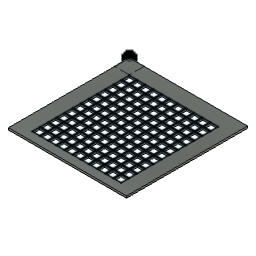
WordClock Raster (Autodesk Fusion 360 design; units mm, degrees)
Autodesk Fusion 360 part; units mm, degrees
sketch "Skizze1" plane through (0, 0, 0) normal (0, 0, 1) x (1, 0, 0)
  line L0 (-74.7669, 75.1961) -> (165.2331, 75.1961)
  line L1 (165.2331, 75.1961) -> (165.2331, -170.8039)
  line L2 (165.2331, -170.8039) -> (-74.7669, -170.8039)
  line L3 (-74.7669, -170.8039) -> (-74.7669, 75.1961)
  dimension "d1" = 240
  dimension "d2" = 246
  constraint horizontal L0
  constraint vertical L1
  constraint horizontal L2
  constraint vertical L3
  measures "d1" distance of L0.start L0.end
  measures "d2" distance of L0.start L2.end
extrude "Extrusion1" add sketch "Skizze1" along normal blind 4
sketch "Skizze2" plane through (0, 0, 4) normal (0, 0, 1) x (-1, 0, 0)
  line L0 (74.7669, 170.8039) -> (-165.2331, 170.8039)
  line L1 (-165.2331, 170.8039) -> (-165.2331, -75.1961)
  line L2 (-165.2331, -75.1961) -> (74.7669, -75.1961)
  line L3 (74.7669, -75.1961) -> (74.7669, 170.8039)
  line L4 (74.7669, -75.1961) -> (44.7989, -75.1961) construction
  line L5 (44.7989, -75.1961) -> (44.7989, -44.9311) construction
  line L6 (44.7989, -44.9311) -> (74.7669, -44.9311) construction
  line L7 (74.7669, -44.9311) -> (74.7669, -75.1961) construction
  line L8 (44.7989, -44.9311) -> (43.7989, -44.9311) construction
  line L9 (43.7989, -44.9311) -> (43.7989, -43.9311) construction
  line L10 (43.7989, -43.9311) -> (44.7989, -43.9311) construction
  line L11 (44.7989, -43.9311) -> (44.7989, -44.9311) construction
  line L12 (43.7989, -43.9311) -> (29.1989, -43.9311)
  line L13 (29.1989, -43.9311) -> (29.1989, -29.3311)
  line L14 (29.1989, -29.3311) -> (43.7989, -29.3311)
  line L15 (43.7989, -29.3311) -> (43.7989, -43.9311)
  line L16 (12.5989, -43.9311) -> (12.5989, -29.3311)
  line L17 (12.5989, -29.3311) -> (27.1989, -29.3311)
  line L18 (27.1989, -29.3311) -> (27.1989, -43.9311)
  line L19 (27.1989, -43.9311) -> (12.5989, -43.9311)
  line L20 (-4.0011, -43.9311) -> (-4.0011, -29.3311)
  line L21 (-4.0011, -29.3311) -> (10.5989, -29.3311)
  line L22 (10.5989, -29.3311) -> (10.5989, -43.9311)
  line L23 (10.5989, -43.9311) -> (-4.0011, -43.9311)
  line L24 (-20.6011, -43.9311) -> (-20.6011, -29.3311)
  line L25 (-20.6011, -29.3311) -> (-6.0011, -29.3311)
  line L26 (-6.0011, -29.3311) -> (-6.0011, -43.9311)
  line L27 (-6.0011, -43.9311) -> (-20.6011, -43.9311)
  line L28 (-37.2011, -43.9311) -> (-37.2011, -29.3311)
  line L29 (-37.2011, -29.3311) -> (-22.6011, -29.3311)
  line L30 (-22.6011, -29.3311) -> (-22.6011, -43.9311)
  line L31 (-22.6011, -43.9311) -> (-37.2011, -43.9311)
  line L32 (-53.8011, -43.9311) -> (-53.8011, -29.3311)
  line L33 (-53.8011, -29.3311) -> (-39.2011, -29.3311)
  line L34 (-39.2011, -29.3311) -> (-39.2011, -43.9311)
  line L35 (-39.2011, -43.9311) -> (-53.8011, -43.9311)
  line L36 (-70.4011, -43.9311) -> (-70.4011, -29.3311)
  line L37 (-70.4011, -29.3311) -> (-55.8011, -29.3311)
  line L38 (-55.8011, -29.3311) -> (-55.8011, -43.9311)
  line L39 (-55.8011, -43.9311) -> (-70.4011, -43.9311)
  line L40 (-87.0011, -43.9311) -> (-87.0011, -29.3311)
  line L41 (-87.0011, -29.3311) -> (-72.4011, -29.3311)
  line L42 (-72.4011, -29.3311) -> (-72.4011, -43.9311)
  line L43 (-72.4011, -43.9311) -> (-87.0011, -43.9311)
  line L44 (-103.6011, -43.9311) -> (-103.6011, -29.3311)
  line L45 (-103.6011, -29.3311) -> (-89.0011, -29.3311)
  line L46 (-89.0011, -29.3311) -> (-89.0011, -43.9311)
  line L47 (-89.0011, -43.9311) -> (-103.6011, -43.9311)
  line L48 (-120.2011, -43.9311) -> (-120.2011, -29.3311)
  line L49 (-120.2011, -29.3311) -> (-105.6011, -29.3311)
  line L50 (-105.6011, -29.3311) -> (-105.6011, -43.9311)
  line L51 (-105.6011, -43.9311) -> (-120.2011, -43.9311)
  line L52 (-136.8011, -43.9311) -> (-136.8011, -29.3311)
  line L53 (-136.8011, -29.3311) -> (-122.2011, -29.3311)
  line L54 (-122.2011, -29.3311) -> (-122.2011, -43.9311)
  line L55 (-122.2011, -43.9311) -> (-136.8011, -43.9311)
  line L56 (29.1989, -27.3311) -> (29.1989, -12.7311)
  line L57 (29.1989, -12.7311) -> (43.7989, -12.7311)
  line L58 (43.7989, -12.7311) -> (43.7989, -27.3311)
  line L59 (43.7989, -27.3311) -> (29.1989, -27.3311)
  line L60 (27.1989, -27.3311) -> (12.5989, -27.3311)
  line L61 (27.1989, -12.7311) -> (27.1989, -27.3311)
  line L62 (12.5989, -12.7311) -> (27.1989, -12.7311)
  line L63 (12.5989, -27.3311) -> (12.5989, -12.7311)
  line L64 (10.5989, -27.3311) -> (-4.0011, -27.3311)
  line L65 (10.5989, -12.7311) -> (10.5989, -27.3311)
  line L66 (-4.0011, -12.7311) -> (10.5989, -12.7311)
  line L67 (-4.0011, -27.3311) -> (-4.0011, -12.7311)
  line L68 (-6.0011, -27.3311) -> (-20.6011, -27.3311)
  line L69 (-6.0011, -12.7311) -> (-6.0011, -27.3311)
  line L70 (-20.6011, -12.7311) -> (-6.0011, -12.7311)
  line L71 (-20.6011, -27.3311) -> (-20.6011, -12.7311)
  line L72 (-22.6011, -27.3311) -> (-37.2011, -27.3311)
  line L73 (-22.6011, -12.7311) -> (-22.6011, -27.3311)
  line L74 (-37.2011, -12.7311) -> (-22.6011, -12.7311)
  line L75 (-37.2011, -27.3311) -> (-37.2011, -12.7311)
  line L76 (-39.2011, -27.3311) -> (-53.8011, -27.3311)
  line L77 (-39.2011, -12.7311) -> (-39.2011, -27.3311)
  line L78 (-53.8011, -12.7311) -> (-39.2011, -12.7311)
  line L79 (-53.8011, -27.3311) -> (-53.8011, -12.7311)
  line L80 (-55.8011, -27.3311) -> (-70.4011, -27.3311)
  line L81 (-55.8011, -12.7311) -> (-55.8011, -27.3311)
  line L82 (-70.4011, -12.7311) -> (-55.8011, -12.7311)
  line L83 (-70.4011, -27.3311) -> (-70.4011, -12.7311)
  line L84 (-72.4011, -27.3311) -> (-87.0011, -27.3311)
  line L85 (-87.0011, -27.3311) -> (-87.0011, -12.7311)
  line L86 (-87.0011, -12.7311) -> (-72.4011, -12.7311)
  line L87 (-72.4011, -12.7311) -> (-72.4011, -27.3311)
  line L88 (-89.0011, -27.3311) -> (-103.6011, -27.3311)
  line L89 (-103.6011, -27.3311) -> (-103.6011, -12.7311)
  line L90 (-103.6011, -12.7311) -> (-89.0011, -12.7311)
  line L91 (-89.0011, -12.7311) -> (-89.0011, -27.3311)
  line L92 (-105.6011, -27.3311) -> (-120.2011, -27.3311)
  line L93 (-120.2011, -27.3311) -> (-120.2011, -12.7311)
  line L94 (-120.2011, -12.7311) -> (-105.6011, -12.7311)
  line L95 (-105.6011, -12.7311) -> (-105.6011, -27.3311)
  line L96 (-122.2011, -27.3311) -> (-136.8011, -27.3311)
  line L97 (-136.8011, -27.3311) -> (-136.8011, -12.7311)
  line L98 (-136.8011, -12.7311) -> (-122.2011, -12.7311)
  line L99 (-122.2011, -12.7311) -> (-122.2011, -27.3311)
  line L100 (29.1989, -10.7311) -> (29.1989, 3.8689)
  line L101 (29.1989, 3.8689) -> (43.7989, 3.8689)
  line L102 (43.7989, 3.8689) -> (43.7989, -10.7311)
  line L103 (43.7989, -10.7311) -> (29.1989, -10.7311)
  line L104 (27.1989, -10.7311) -> (12.5989, -10.7311)
  line L105 (27.1989, 3.8689) -> (27.1989, -10.7311)
  line L106 (12.5989, 3.8689) -> (27.1989, 3.8689)
  line L107 (12.5989, -10.7311) -> (12.5989, 3.8689)
  line L108 (10.5989, -10.7311) -> (-4.0011, -10.7311)
  line L109 (10.5989, 3.8689) -> (10.5989, -10.7311)
  line L110 (-4.0011, 3.8689) -> (10.5989, 3.8689)
  line L111 (-4.0011, -10.7311) -> (-4.0011, 3.8689)
  line L112 (-6.0011, -10.7311) -> (-20.6011, -10.7311)
  line L113 (-6.0011, 3.8689) -> (-6.0011, -10.7311)
  line L114 (-20.6011, 3.8689) -> (-6.0011, 3.8689)
  line L115 (-20.6011, -10.7311) -> (-20.6011, 3.8689)
  line L116 (-22.6011, -10.7311) -> (-37.2011, -10.7311)
  line L117 (-22.6011, 3.8689) -> (-22.6011, -10.7311)
  line L118 (-37.2011, 3.8689) -> (-22.6011, 3.8689)
  line L119 (-37.2011, -10.7311) -> (-37.2011, 3.8689)
  line L120 (-39.2011, -10.7311) -> (-53.8011, -10.7311)
  line L121 (-39.2011, 3.8689) -> (-39.2011, -10.7311)
  line L122 (-53.8011, 3.8689) -> (-39.2011, 3.8689)
  line L123 (-53.8011, -10.7311) -> (-53.8011, 3.8689)
  line L124 (-55.8011, -10.7311) -> (-70.4011, -10.7311)
  line L125 (-55.8011, 3.8689) -> (-55.8011, -10.7311)
  line L126 (-70.4011, 3.8689) -> (-55.8011, 3.8689)
  line L127 (-70.4011, -10.7311) -> (-70.4011, 3.8689)
  line L128 (-72.4011, -10.7311) -> (-87.0011, -10.7311)
  line L129 (-87.0011, -10.7311) -> (-87.0011, 3.8689)
  line L130 (-87.0011, 3.8689) -> (-72.4011, 3.8689)
  line L131 (-72.4011, 3.8689) -> (-72.4011, -10.7311)
  line L132 (-89.0011, -10.7311) -> (-103.6011, -10.7311)
  line L133 (-103.6011, -10.7311) -> (-103.6011, 3.8689)
  line L134 (-103.6011, 3.8689) -> (-89.0011, 3.8689)
  line L135 (-89.0011, 3.8689) -> (-89.0011, -10.7311)
  line L136 (-105.6011, -10.7311) -> (-120.2011, -10.7311)
  line L137 (-120.2011, -10.7311) -> (-120.2011, 3.8689)
  line L138 (-120.2011, 3.8689) -> (-105.6011, 3.8689)
  line L139 (-105.6011, 3.8689) -> (-105.6011, -10.7311)
  line L140 (-122.2011, -10.7311) -> (-136.8011, -10.7311)
  line L141 (-136.8011, -10.7311) -> (-136.8011, 3.8689)
  line L142 (-136.8011, 3.8689) -> (-122.2011, 3.8689)
  line L143 (-122.2011, 3.8689) -> (-122.2011, -10.7311)
  line L144 (29.1989, 5.8689) -> (29.1989, 20.4689)
  line L145 (29.1989, 20.4689) -> (43.7989, 20.4689)
  line L146 (43.7989, 20.4689) -> (43.7989, 5.8689)
  line L147 (43.7989, 5.8689) -> (29.1989, 5.8689)
  line L148 (27.1989, 5.8689) -> (12.5989, 5.8689)
  line L149 (27.1989, 20.4689) -> (27.1989, 5.8689)
  line L150 (12.5989, 20.4689) -> (27.1989, 20.4689)
  line L151 (12.5989, 5.8689) -> (12.5989, 20.4689)
  line L152 (10.5989, 5.8689) -> (-4.0011, 5.8689)
  line L153 (10.5989, 20.4689) -> (10.5989, 5.8689)
  line L154 (-4.0011, 20.4689) -> (10.5989, 20.4689)
  line L155 (-4.0011, 5.8689) -> (-4.0011, 20.4689)
  line L156 (-6.0011, 5.8689) -> (-20.6011, 5.8689)
  line L157 (-6.0011, 20.4689) -> (-6.0011, 5.8689)
  line L158 (-20.6011, 20.4689) -> (-6.0011, 20.4689)
  line L159 (-20.6011, 5.8689) -> (-20.6011, 20.4689)
  line L160 (-22.6011, 5.8689) -> (-37.2011, 5.8689)
  line L161 (-22.6011, 20.4689) -> (-22.6011, 5.8689)
  line L162 (-37.2011, 20.4689) -> (-22.6011, 20.4689)
  line L163 (-37.2011, 5.8689) -> (-37.2011, 20.4689)
  line L164 (-39.2011, 5.8689) -> (-53.8011, 5.8689)
  line L165 (-39.2011, 20.4689) -> (-39.2011, 5.8689)
  line L166 (-53.8011, 20.4689) -> (-39.2011, 20.4689)
  line L167 (-53.8011, 5.8689) -> (-53.8011, 20.4689)
  line L168 (-55.8011, 5.8689) -> (-70.4011, 5.8689)
  line L169 (-55.8011, 20.4689) -> (-55.8011, 5.8689)
  line L170 (-70.4011, 20.4689) -> (-55.8011, 20.4689)
  line L171 (-70.4011, 5.8689) -> (-70.4011, 20.4689)
  line L172 (-72.4011, 5.8689) -> (-87.0011, 5.8689)
  line L173 (-87.0011, 5.8689) -> (-87.0011, 20.4689)
  line L174 (-87.0011, 20.4689) -> (-72.4011, 20.4689)
  line L175 (-72.4011, 20.4689) -> (-72.4011, 5.8689)
  line L176 (-89.0011, 5.8689) -> (-103.6011, 5.8689)
  line L177 (-103.6011, 5.8689) -> (-103.6011, 20.4689)
  line L178 (-103.6011, 20.4689) -> (-89.0011, 20.4689)
  line L179 (-89.0011, 20.4689) -> (-89.0011, 5.8689)
  line L180 (-105.6011, 5.8689) -> (-120.2011, 5.8689)
  line L181 (-120.2011, 5.8689) -> (-120.2011, 20.4689)
  line L182 (-120.2011, 20.4689) -> (-105.6011, 20.4689)
  line L183 (-105.6011, 20.4689) -> (-105.6011, 5.8689)
  line L184 (-122.2011, 5.8689) -> (-136.8011, 5.8689)
  line L185 (-136.8011, 5.8689) -> (-136.8011, 20.4689)
  line L186 (-136.8011, 20.4689) -> (-122.2011, 20.4689)
  line L187 (-122.2011, 20.4689) -> (-122.2011, 5.8689)
  line L188 (29.1989, 22.4689) -> (29.1989, 37.0689)
  line L189 (29.1989, 37.0689) -> (43.7989, 37.0689)
  line L190 (43.7989, 37.0689) -> (43.7989, 22.4689)
  line L191 (43.7989, 22.4689) -> (29.1989, 22.4689)
  line L192 (27.1989, 22.4689) -> (12.5989, 22.4689)
  line L193 (27.1989, 37.0689) -> (27.1989, 22.4689)
  line L194 (12.5989, 37.0689) -> (27.1989, 37.0689)
  line L195 (12.5989, 22.4689) -> (12.5989, 37.0689)
  line L196 (10.5989, 22.4689) -> (-4.0011, 22.4689)
  line L197 (10.5989, 37.0689) -> (10.5989, 22.4689)
  line L198 (-4.0011, 37.0689) -> (10.5989, 37.0689)
  line L199 (-4.0011, 22.4689) -> (-4.0011, 37.0689)
  line L200 (-6.0011, 22.4689) -> (-20.6011, 22.4689)
  line L201 (-6.0011, 37.0689) -> (-6.0011, 22.4689)
  line L202 (-20.6011, 37.0689) -> (-6.0011, 37.0689)
  line L203 (-20.6011, 22.4689) -> (-20.6011, 37.0689)
  line L204 (-22.6011, 22.4689) -> (-37.2011, 22.4689)
  line L205 (-22.6011, 37.0689) -> (-22.6011, 22.4689)
  line L206 (-37.2011, 37.0689) -> (-22.6011, 37.0689)
  line L207 (-37.2011, 22.4689) -> (-37.2011, 37.0689)
  line L208 (-39.2011, 22.4689) -> (-53.8011, 22.4689)
  line L209 (-39.2011, 37.0689) -> (-39.2011, 22.4689)
  line L210 (-53.8011, 37.0689) -> (-39.2011, 37.0689)
  line L211 (-53.8011, 22.4689) -> (-53.8011, 37.0689)
  line L212 (-55.8011, 22.4689) -> (-70.4011, 22.4689)
  line L213 (-55.8011, 37.0689) -> (-55.8011, 22.4689)
  line L214 (-70.4011, 37.0689) -> (-55.8011, 37.0689)
  line L215 (-70.4011, 22.4689) -> (-70.4011, 37.0689)
  line L216 (-72.4011, 22.4689) -> (-87.0011, 22.4689)
  line L217 (-87.0011, 22.4689) -> (-87.0011, 37.0689)
  line L218 (-87.0011, 37.0689) -> (-72.4011, 37.0689)
  line L219 (-72.4011, 37.0689) -> (-72.4011, 22.4689)
  line L220 (-89.0011, 22.4689) -> (-103.6011, 22.4689)
  line L221 (-103.6011, 22.4689) -> (-103.6011, 37.0689)
  line L222 (-103.6011, 37.0689) -> (-89.0011, 37.0689)
  line L223 (-89.0011, 37.0689) -> (-89.0011, 22.4689)
  line L224 (-105.6011, 22.4689) -> (-120.2011, 22.4689)
  line L225 (-120.2011, 22.4689) -> (-120.2011, 37.0689)
  line L226 (-120.2011, 37.0689) -> (-105.6011, 37.0689)
  line L227 (-105.6011, 37.0689) -> (-105.6011, 22.4689)
  line L228 (-122.2011, 22.4689) -> (-136.8011, 22.4689)
  line L229 (-136.8011, 22.4689) -> (-136.8011, 37.0689)
  line L230 (-136.8011, 37.0689) -> (-122.2011, 37.0689)
  line L231 (-122.2011, 37.0689) -> (-122.2011, 22.4689)
  line L232 (29.1989, 39.0689) -> (29.1989, 53.6689)
  line L233 (29.1989, 53.6689) -> (43.7989, 53.6689)
  line L234 (43.7989, 53.6689) -> (43.7989, 39.0689)
  line L235 (43.7989, 39.0689) -> (29.1989, 39.0689)
  line L236 (27.1989, 39.0689) -> (12.5989, 39.0689)
  line L237 (27.1989, 53.6689) -> (27.1989, 39.0689)
  line L238 (12.5989, 53.6689) -> (27.1989, 53.6689)
  line L239 (12.5989, 39.0689) -> (12.5989, 53.6689)
  line L240 (10.5989, 39.0689) -> (-4.0011, 39.0689)
  line L241 (10.5989, 53.6689) -> (10.5989, 39.0689)
  line L242 (-4.0011, 53.6689) -> (10.5989, 53.6689)
  line L243 (-4.0011, 39.0689) -> (-4.0011, 53.6689)
  line L244 (-6.0011, 39.0689) -> (-20.6011, 39.0689)
  line L245 (-6.0011, 53.6689) -> (-6.0011, 39.0689)
  line L246 (-20.6011, 53.6689) -> (-6.0011, 53.6689)
  line L247 (-20.6011, 39.0689) -> (-20.6011, 53.6689)
  line L248 (-22.6011, 39.0689) -> (-37.2011, 39.0689)
  line L249 (-22.6011, 53.6689) -> (-22.6011, 39.0689)
  line L250 (-37.2011, 53.6689) -> (-22.6011, 53.6689)
  line L251 (-37.2011, 39.0689) -> (-37.2011, 53.6689)
  line L252 (-39.2011, 39.0689) -> (-53.8011, 39.0689)
  line L253 (-39.2011, 53.6689) -> (-39.2011, 39.0689)
  line L254 (-53.8011, 53.6689) -> (-39.2011, 53.6689)
  line L255 (-53.8011, 39.0689) -> (-53.8011, 53.6689)
  line L256 (-55.8011, 39.0689) -> (-70.4011, 39.0689)
  line L257 (-55.8011, 53.6689) -> (-55.8011, 39.0689)
  line L258 (-70.4011, 53.6689) -> (-55.8011, 53.6689)
  line L259 (-70.4011, 39.0689) -> (-70.4011, 53.6689)
  line L260 (-72.4011, 39.0689) -> (-87.0011, 39.0689)
  line L261 (-87.0011, 39.0689) -> (-87.0011, 53.6689)
  line L262 (-87.0011, 53.6689) -> (-72.4011, 53.6689)
  line L263 (-72.4011, 53.6689) -> (-72.4011, 39.0689)
  line L264 (-89.0011, 39.0689) -> (-103.6011, 39.0689)
  line L265 (-103.6011, 39.0689) -> (-103.6011, 53.6689)
  line L266 (-103.6011, 53.6689) -> (-89.0011, 53.6689)
  line L267 (-89.0011, 53.6689) -> (-89.0011, 39.0689)
  line L268 (-105.6011, 39.0689) -> (-120.2011, 39.0689)
  line L269 (-120.2011, 39.0689) -> (-120.2011, 53.6689)
  line L270 (-120.2011, 53.6689) -> (-105.6011, 53.6689)
  line L271 (-105.6011, 53.6689) -> (-105.6011, 39.0689)
  line L272 (-122.2011, 39.0689) -> (-136.8011, 39.0689)
  line L273 (-136.8011, 39.0689) -> (-136.8011, 53.6689)
  line L274 (-136.8011, 53.6689) -> (-122.2011, 53.6689)
  line L275 (-122.2011, 53.6689) -> (-122.2011, 39.0689)
  line L276 (29.1989, 55.6689) -> (29.1989, 70.2689)
  line L277 (29.1989, 70.2689) -> (43.7989, 70.2689)
  line L278 (43.7989, 70.2689) -> (43.7989, 55.6689)
  line L279 (43.7989, 55.6689) -> (29.1989, 55.6689)
  line L280 (27.1989, 55.6689) -> (12.5989, 55.6689)
  line L281 (27.1989, 70.2689) -> (27.1989, 55.6689)
  line L282 (12.5989, 70.2689) -> (27.1989, 70.2689)
  line L283 (12.5989, 55.6689) -> (12.5989, 70.2689)
  line L284 (10.5989, 55.6689) -> (-4.0011, 55.6689)
  line L285 (10.5989, 70.2689) -> (10.5989, 55.6689)
  line L286 (-4.0011, 70.2689) -> (10.5989, 70.2689)
  line L287 (-4.0011, 55.6689) -> (-4.0011, 70.2689)
  line L288 (-6.0011, 55.6689) -> (-20.6011, 55.6689)
  line L289 (-6.0011, 70.2689) -> (-6.0011, 55.6689)
  line L290 (-20.6011, 70.2689) -> (-6.0011, 70.2689)
  line L291 (-20.6011, 55.6689) -> (-20.6011, 70.2689)
  line L292 (-22.6011, 55.6689) -> (-37.2011, 55.6689)
  line L293 (-22.6011, 70.2689) -> (-22.6011, 55.6689)
  line L294 (-37.2011, 70.2689) -> (-22.6011, 70.2689)
  line L295 (-37.2011, 55.6689) -> (-37.2011, 70.2689)
  line L296 (-39.2011, 55.6689) -> (-53.8011, 55.6689)
  line L297 (-39.2011, 70.2689) -> (-39.2011, 55.6689)
  line L298 (-53.8011, 70.2689) -> (-39.2011, 70.2689)
  line L299 (-53.8011, 55.6689) -> (-53.8011, 70.2689)
  line L300 (-55.8011, 55.6689) -> (-70.4011, 55.6689)
  line L301 (-55.8011, 70.2689) -> (-55.8011, 55.6689)
  line L302 (-70.4011, 70.2689) -> (-55.8011, 70.2689)
  line L303 (-70.4011, 55.6689) -> (-70.4011, 70.2689)
  line L304 (-72.4011, 55.6689) -> (-87.0011, 55.6689)
  line L305 (-87.0011, 55.6689) -> (-87.0011, 70.2689)
  line L306 (-87.0011, 70.2689) -> (-72.4011, 70.2689)
  line L307 (-72.4011, 70.2689) -> (-72.4011, 55.6689)
  line L308 (-89.0011, 55.6689) -> (-103.6011, 55.6689)
  line L309 (-103.6011, 55.6689) -> (-103.6011, 70.2689)
  line L310 (-103.6011, 70.2689) -> (-89.0011, 70.2689)
  line L311 (-89.0011, 70.2689) -> (-89.0011, 55.6689)
  line L312 (-105.6011, 55.6689) -> (-120.2011, 55.6689)
  line L313 (-120.2011, 55.6689) -> (-120.2011, 70.2689)
  line L314 (-120.2011, 70.2689) -> (-105.6011, 70.2689)
  line L315 (-105.6011, 70.2689) -> (-105.6011, 55.6689)
  line L316 (-122.2011, 55.6689) -> (-136.8011, 55.6689)
  line L317 (-136.8011, 55.6689) -> (-136.8011, 70.2689)
  line L318 (-136.8011, 70.2689) -> (-122.2011, 70.2689)
  line L319 (-122.2011, 70.2689) -> (-122.2011, 55.6689)
  line L320 (29.1989, 72.2689) -> (29.1989, 86.8689)
  line L321 (29.1989, 86.8689) -> (43.7989, 86.8689)
  line L322 (43.7989, 86.8689) -> (43.7989, 72.2689)
  line L323 (43.7989, 72.2689) -> (29.1989, 72.2689)
  line L324 (27.1989, 72.2689) -> (12.5989, 72.2689)
  line L325 (27.1989, 86.8689) -> (27.1989, 72.2689)
  line L326 (12.5989, 86.8689) -> (27.1989, 86.8689)
  line L327 (12.5989, 72.2689) -> (12.5989, 86.8689)
  line L328 (10.5989, 72.2689) -> (-4.0011, 72.2689)
  line L329 (10.5989, 86.8689) -> (10.5989, 72.2689)
  line L330 (-4.0011, 86.8689) -> (10.5989, 86.8689)
  line L331 (-4.0011, 72.2689) -> (-4.0011, 86.8689)
  line L332 (-6.0011, 72.2689) -> (-20.6011, 72.2689)
  line L333 (-6.0011, 86.8689) -> (-6.0011, 72.2689)
  line L334 (-20.6011, 86.8689) -> (-6.0011, 86.8689)
  line L335 (-20.6011, 72.2689) -> (-20.6011, 86.8689)
  line L336 (-22.6011, 72.2689) -> (-37.2011, 72.2689)
  line L337 (-22.6011, 86.8689) -> (-22.6011, 72.2689)
  line L338 (-37.2011, 86.8689) -> (-22.6011, 86.8689)
  line L339 (-37.2011, 72.2689) -> (-37.2011, 86.8689)
  line L340 (-39.2011, 72.2689) -> (-53.8011, 72.2689)
  line L341 (-39.2011, 86.8689) -> (-39.2011, 72.2689)
  line L342 (-53.8011, 86.8689) -> (-39.2011, 86.8689)
  line L343 (-53.8011, 72.2689) -> (-53.8011, 86.8689)
  line L344 (-55.8011, 72.2689) -> (-70.4011, 72.2689)
  line L345 (-55.8011, 86.8689) -> (-55.8011, 72.2689)
  line L346 (-70.4011, 86.8689) -> (-55.8011, 86.8689)
  line L347 (-70.4011, 72.2689) -> (-70.4011, 86.8689)
  line L348 (-72.4011, 72.2689) -> (-87.0011, 72.2689)
  line L349 (-87.0011, 72.2689) -> (-87.0011, 86.8689)
  line L350 (-87.0011, 86.8689) -> (-72.4011, 86.8689)
  line L351 (-72.4011, 86.8689) -> (-72.4011, 72.2689)
  line L352 (-89.0011, 72.2689) -> (-103.6011, 72.2689)
  line L353 (-103.6011, 72.2689) -> (-103.6011, 86.8689)
  line L354 (-103.6011, 86.8689) -> (-89.0011, 86.8689)
  line L355 (-89.0011, 86.8689) -> (-89.0011, 72.2689)
  line L356 (-105.6011, 72.2689) -> (-120.2011, 72.2689)
  line L357 (-120.2011, 72.2689) -> (-120.2011, 86.8689)
  line L358 (-120.2011, 86.8689) -> (-105.6011, 86.8689)
  line L359 (-105.6011, 86.8689) -> (-105.6011, 72.2689)
  line L360 (-122.2011, 72.2689) -> (-136.8011, 72.2689)
  line L361 (-136.8011, 72.2689) -> (-136.8011, 86.8689)
  line L362 (-136.8011, 86.8689) -> (-122.2011, 86.8689)
  line L363 (-122.2011, 86.8689) -> (-122.2011, 72.2689)
  line L364 (29.1989, 88.8689) -> (29.1989, 103.4689)
  line L365 (29.1989, 103.4689) -> (43.7989, 103.4689)
  line L366 (43.7989, 103.4689) -> (43.7989, 88.8689)
  line L367 (43.7989, 88.8689) -> (29.1989, 88.8689)
  line L368 (27.1989, 88.8689) -> (12.5989, 88.8689)
  line L369 (27.1989, 103.4689) -> (27.1989, 88.8689)
  line L370 (12.5989, 103.4689) -> (27.1989, 103.4689)
  line L371 (12.5989, 88.8689) -> (12.5989, 103.4689)
  line L372 (10.5989, 88.8689) -> (-4.0011, 88.8689)
  line L373 (10.5989, 103.4689) -> (10.5989, 88.8689)
  line L374 (-4.0011, 103.4689) -> (10.5989, 103.4689)
  line L375 (-4.0011, 88.8689) -> (-4.0011, 103.4689)
  line L376 (-6.0011, 88.8689) -> (-20.6011, 88.8689)
  line L377 (-6.0011, 103.4689) -> (-6.0011, 88.8689)
  line L378 (-20.6011, 103.4689) -> (-6.0011, 103.4689)
  line L379 (-20.6011, 88.8689) -> (-20.6011, 103.4689)
  line L380 (-22.6011, 88.8689) -> (-37.2011, 88.8689)
  line L381 (-22.6011, 103.4689) -> (-22.6011, 88.8689)
  line L382 (-37.2011, 103.4689) -> (-22.6011, 103.4689)
  line L383 (-37.2011, 88.8689) -> (-37.2011, 103.4689)
  line L384 (-39.2011, 88.8689) -> (-53.8011, 88.8689)
  line L385 (-39.2011, 103.4689) -> (-39.2011, 88.8689)
  line L386 (-53.8011, 103.4689) -> (-39.2011, 103.4689)
  line L387 (-53.8011, 88.8689) -> (-53.8011, 103.4689)
  line L388 (-55.8011, 88.8689) -> (-70.4011, 88.8689)
  line L389 (-55.8011, 103.4689) -> (-55.8011, 88.8689)
  line L390 (-70.4011, 103.4689) -> (-55.8011, 103.4689)
  line L391 (-70.4011, 88.8689) -> (-70.4011, 103.4689)
  line L392 (-72.4011, 88.8689) -> (-87.0011, 88.8689)
  line L393 (-87.0011, 88.8689) -> (-87.0011, 103.4689)
  line L394 (-87.0011, 103.4689) -> (-72.4011, 103.4689)
  line L395 (-72.4011, 103.4689) -> (-72.4011, 88.8689)
  line L396 (-89.0011, 88.8689) -> (-103.6011, 88.8689)
  line L397 (-103.6011, 88.8689) -> (-103.6011, 103.4689)
  line L398 (-103.6011, 103.4689) -> (-89.0011, 103.4689)
  line L399 (-89.0011, 103.4689) -> (-89.0011, 88.8689)
  line L400 (-105.6011, 88.8689) -> (-120.2011, 88.8689)
  line L401 (-120.2011, 88.8689) -> (-120.2011, 103.4689)
  line L402 (-120.2011, 103.4689) -> (-105.6011, 103.4689)
  line L403 (-105.6011, 103.4689) -> (-105.6011, 88.8689)
  line L404 (-122.2011, 88.8689) -> (-136.8011, 88.8689)
  line L405 (-136.8011, 88.8689) -> (-136.8011, 103.4689)
  line L406 (-136.8011, 103.4689) -> (-122.2011, 103.4689)
  line L407 (-122.2011, 103.4689) -> (-122.2011, 88.8689)
  line L408 (29.1989, 105.4689) -> (29.1989, 120.0689)
  line L409 (29.1989, 120.0689) -> (43.7989, 120.0689)
  line L410 (43.7989, 120.0689) -> (43.7989, 105.4689)
  line L411 (43.7989, 105.4689) -> (29.1989, 105.4689)
  line L412 (27.1989, 105.4689) -> (12.5989, 105.4689)
  line L413 (27.1989, 120.0689) -> (27.1989, 105.4689)
  line L414 (12.5989, 120.0689) -> (27.1989, 120.0689)
  line L415 (12.5989, 105.4689) -> (12.5989, 120.0689)
  line L416 (10.5989, 105.4689) -> (-4.0011, 105.4689)
  line L417 (10.5989, 120.0689) -> (10.5989, 105.4689)
  line L418 (-4.0011, 120.0689) -> (10.5989, 120.0689)
  line L419 (-4.0011, 105.4689) -> (-4.0011, 120.0689)
  line L420 (-6.0011, 105.4689) -> (-20.6011, 105.4689)
  line L421 (-6.0011, 120.0689) -> (-6.0011, 105.4689)
  line L422 (-20.6011, 120.0689) -> (-6.0011, 120.0689)
  line L423 (-20.6011, 105.4689) -> (-20.6011, 120.0689)
  line L424 (-22.6011, 105.4689) -> (-37.2011, 105.4689)
  line L425 (-22.6011, 120.0689) -> (-22.6011, 105.4689)
  line L426 (-37.2011, 120.0689) -> (-22.6011, 120.0689)
  line L427 (-37.2011, 105.4689) -> (-37.2011, 120.0689)
  line L428 (-39.2011, 105.4689) -> (-53.8011, 105.4689)
  line L429 (-39.2011, 120.0689) -> (-39.2011, 105.4689)
  line L430 (-53.8011, 120.0689) -> (-39.2011, 120.0689)
  line L431 (-53.8011, 105.4689) -> (-53.8011, 120.0689)
  line L432 (-55.8011, 105.4689) -> (-70.4011, 105.4689)
  line L433 (-55.8011, 120.0689) -> (-55.8011, 105.4689)
  line L434 (-70.4011, 120.0689) -> (-55.8011, 120.0689)
  line L435 (-70.4011, 105.4689) -> (-70.4011, 120.0689)
  line L436 (-72.4011, 105.4689) -> (-87.0011, 105.4689)
  line L437 (-87.0011, 105.4689) -> (-87.0011, 120.0689)
  line L438 (-87.0011, 120.0689) -> (-72.4011, 120.0689)
  line L439 (-72.4011, 120.0689) -> (-72.4011, 105.4689)
  line L440 (-89.0011, 105.4689) -> (-103.6011, 105.4689)
  line L441 (-103.6011, 105.4689) -> (-103.6011, 120.0689)
  line L442 (-103.6011, 120.0689) -> (-89.0011, 120.0689)
  line L443 (-89.0011, 120.0689) -> (-89.0011, 105.4689)
  line L444 (-105.6011, 105.4689) -> (-120.2011, 105.4689)
  line L445 (-120.2011, 105.4689) -> (-120.2011, 120.0689)
  line L446 (-120.2011, 120.0689) -> (-105.6011, 120.0689)
  line L447 (-105.6011, 120.0689) -> (-105.6011, 105.4689)
  line L448 (-122.2011, 105.4689) -> (-136.8011, 105.4689)
  line L449 (-136.8011, 105.4689) -> (-136.8011, 120.0689)
  line L450 (-136.8011, 120.0689) -> (-122.2011, 120.0689)
  line L451 (-122.2011, 120.0689) -> (-122.2011, 105.4689)
  line L452 (29.1989, 122.0689) -> (29.1989, 136.6689)
  line L453 (29.1989, 136.6689) -> (43.7989, 136.6689)
  line L454 (43.7989, 136.6689) -> (43.7989, 122.0689)
  line L455 (43.7989, 122.0689) -> (29.1989, 122.0689)
  line L456 (27.1989, 122.0689) -> (12.5989, 122.0689)
  line L457 (27.1989, 136.6689) -> (27.1989, 122.0689)
  line L458 (12.5989, 136.6689) -> (27.1989, 136.6689)
  line L459 (12.5989, 122.0689) -> (12.5989, 136.6689)
  line L460 (10.5989, 122.0689) -> (-4.0011, 122.0689)
  line L461 (10.5989, 136.6689) -> (10.5989, 122.0689)
  line L462 (-4.0011, 136.6689) -> (10.5989, 136.6689)
  line L463 (-4.0011, 122.0689) -> (-4.0011, 136.6689)
  line L464 (-6.0011, 122.0689) -> (-20.6011, 122.0689)
  line L465 (-6.0011, 136.6689) -> (-6.0011, 122.0689)
  line L466 (-20.6011, 136.6689) -> (-6.0011, 136.6689)
  line L467 (-20.6011, 122.0689) -> (-20.6011, 136.6689)
  line L468 (-22.6011, 122.0689) -> (-37.2011, 122.0689)
  line L469 (-22.6011, 136.6689) -> (-22.6011, 122.0689)
  line L470 (-37.2011, 136.6689) -> (-22.6011, 136.6689)
  line L471 (-37.2011, 122.0689) -> (-37.2011, 136.6689)
  line L472 (-39.2011, 122.0689) -> (-53.8011, 122.0689)
  line L473 (-39.2011, 136.6689) -> (-39.2011, 122.0689)
  line L474 (-53.8011, 136.6689) -> (-39.2011, 136.6689)
  line L475 (-53.8011, 122.0689) -> (-53.8011, 136.6689)
  line L476 (-55.8011, 122.0689) -> (-70.4011, 122.0689)
  line L477 (-55.8011, 136.6689) -> (-55.8011, 122.0689)
  line L478 (-70.4011, 136.6689) -> (-55.8011, 136.6689)
  line L479 (-70.4011, 122.0689) -> (-70.4011, 136.6689)
  line L480 (-72.4011, 122.0689) -> (-87.0011, 122.0689)
  line L481 (-87.0011, 122.0689) -> (-87.0011, 136.6689)
  line L482 (-87.0011, 136.6689) -> (-72.4011, 136.6689)
  line L483 (-72.4011, 136.6689) -> (-72.4011, 122.0689)
  line L484 (-89.0011, 122.0689) -> (-103.6011, 122.0689)
  line L485 (-103.6011, 122.0689) -> (-103.6011, 136.6689)
  line L486 (-103.6011, 136.6689) -> (-89.0011, 136.6689)
  line L487 (-89.0011, 136.6689) -> (-89.0011, 122.0689)
  line L488 (-105.6011, 122.0689) -> (-120.2011, 122.0689)
  line L489 (-120.2011, 122.0689) -> (-120.2011, 136.6689)
  line L490 (-120.2011, 136.6689) -> (-105.6011, 136.6689)
  line L491 (-105.6011, 136.6689) -> (-105.6011, 122.0689)
  line L492 (-122.2011, 122.0689) -> (-136.8011, 122.0689)
  line L493 (-136.8011, 122.0689) -> (-136.8011, 136.6689)
  line L494 (-136.8011, 136.6689) -> (-122.2011, 136.6689)
  line L495 (-122.2011, 136.6689) -> (-122.2011, 122.0689)
  line L496 (29.1989, 138.6689) -> (29.1989, 153.2689)
  line L497 (29.1989, 153.2689) -> (43.7989, 153.2689)
  line L498 (43.7989, 153.2689) -> (43.7989, 138.6689)
  line L499 (43.7989, 138.6689) -> (29.1989, 138.6689)
  line L500 (27.1989, 138.6689) -> (12.5989, 138.6689)
  line L501 (27.1989, 153.2689) -> (27.1989, 138.6689)
  line L502 (12.5989, 153.2689) -> (27.1989, 153.2689)
  line L503 (12.5989, 138.6689) -> (12.5989, 153.2689)
  line L504 (10.5989, 138.6689) -> (-4.0011, 138.6689)
  line L505 (10.5989, 153.2689) -> (10.5989, 138.6689)
  line L506 (-4.0011, 153.2689) -> (10.5989, 153.2689)
  line L507 (-4.0011, 138.6689) -> (-4.0011, 153.2689)
  line L508 (-6.0011, 138.6689) -> (-20.6011, 138.6689)
  line L509 (-6.0011, 153.2689) -> (-6.0011, 138.6689)
  line L510 (-20.6011, 153.2689) -> (-6.0011, 153.2689)
  line L511 (-20.6011, 138.6689) -> (-20.6011, 153.2689)
  line L512 (-22.6011, 138.6689) -> (-37.2011, 138.6689)
  line L513 (-22.6011, 153.2689) -> (-22.6011, 138.6689)
  line L514 (-37.2011, 153.2689) -> (-22.6011, 153.2689)
  line L515 (-37.2011, 138.6689) -> (-37.2011, 153.2689)
  line L516 (-39.2011, 138.6689) -> (-53.8011, 138.6689)
  line L517 (-39.2011, 153.2689) -> (-39.2011, 138.6689)
  line L518 (-53.8011, 153.2689) -> (-39.2011, 153.2689)
  line L519 (-53.8011, 138.6689) -> (-53.8011, 153.2689)
  line L520 (-55.8011, 138.6689) -> (-70.4011, 138.6689)
  line L521 (-55.8011, 153.2689) -> (-55.8011, 138.6689)
  line L522 (-70.4011, 153.2689) -> (-55.8011, 153.2689)
  line L523 (-70.4011, 138.6689) -> (-70.4011, 153.2689)
  line L524 (-72.4011, 138.6689) -> (-87.0011, 138.6689)
  line L525 (-87.0011, 138.6689) -> (-87.0011, 153.2689)
  line L526 (-87.0011, 153.2689) -> (-72.4011, 153.2689)
  line L527 (-72.4011, 153.2689) -> (-72.4011, 138.6689)
  line L528 (-89.0011, 138.6689) -> (-103.6011, 138.6689)
  line L529 (-103.6011, 138.6689) -> (-103.6011, 153.2689)
  line L530 (-103.6011, 153.2689) -> (-89.0011, 153.2689)
  line L531 (-89.0011, 153.2689) -> (-89.0011, 138.6689)
  line L532 (-105.6011, 138.6689) -> (-120.2011, 138.6689)
  line L533 (-120.2011, 138.6689) -> (-120.2011, 153.2689)
  line L534 (-120.2011, 153.2689) -> (-105.6011, 153.2689)
  line L535 (-105.6011, 153.2689) -> (-105.6011, 138.6689)
  line L536 (-122.2011, 138.6689) -> (-136.8011, 138.6689)
  line L537 (-136.8011, 138.6689) -> (-136.8011, 153.2689)
  line L538 (-136.8011, 153.2689) -> (-122.2011, 153.2689)
  line L539 (-122.2011, 153.2689) -> (-122.2011, 138.6689)
  dimension "d5" = 29.968
  dimension "d6" = 30.265
  dimension "d7" = 1
  dimension "d8" = 1
  dimension "d9" = 14.6
  dimension "d10" = 14.6
  dimension "d13" = -166
  dimension "d14" = 0
  dimension "d19" = 0
  dimension "d20" = 182.6
  constraint horizontal L4
  constraint vertical L5
  constraint horizontal L6
  constraint vertical L7
  constraint coincident L2.end L3.start
  constraint horizontal L8
  constraint vertical L9
  constraint horizontal L10
  constraint vertical L11
  constraint horizontal L12
  constraint vertical L13
  constraint horizontal L14
  constraint vertical L15
  measures "d5" distance of L2.end L4.end
  measures "d6" distance of L2.end L6.end
  measures "d7" distance of L5.end L8.end
  measures "d8" distance of L5.end L10.end
  measures "d9" distance of L9.end L12.end
  measures "d10" distance of L9.end L14.end
extrude "Extrusion2" cut sketch "Skizze2" against normal blind 4 contours L12 L13 L14 L15 | L16 L17 L18 L19 | L20 L21 L22 L23 | L24 L25 L26 L27 | L28 L29 L30 L31 | L32 L33 L34 L35 | L36 L37 L38 L39 | L40 L41 L42 L43 | L44 L45 L46 L47 | L48 L49 L50 L51 | L52 L53 L54 L55 | L56 L57 L58 L59 | L60 L61 L62 L63 | L64 L65 L66 L67 | L68 L69 L70 L71 | L72 L73 L74 L75 | L76 L77 L78 L79 | L80 L81 L82 L83 | L84 L85 L86 L87 | L88 L89 L90 L91 | L92 L93 L94 L95 | L96 L97 L98 L99 | L100 L101 L102 L103 | L104 L105 L106 L107 | L108 L109 L110 L111 | L112 L113 L114 L115 | L116 L117 L118 L119 | L120 L121 L122 L123 | L124 L125 L126 L127 | L128 L129 L130 L131 | L132 L133 L134 L135 | L136 L137 L138 L139 | L140 L141 L142 L143 | L144 L145 L146 L147 | L148 L149 L150 L151 | L152 L153 L154 L155 | L156 L157 L158 L159 | L160 L161 L162 L163 | L164 L165 L166 L167 | L168 L169 L170 L171 | L172 L173 L174 L175 | L176 L177 L178 L179 | L180 L181 L182 L183 | L184 L185 L186 L187 | L188 L189 L190 L191 | L192 L193 L194 L195 | L196 L197 L198 L199 | L200 L201 L202 L203 | L204 L205 L206 L207 | L208 L209 L210 L211 | L212 L213 L214 L215 | L216 L217 L218 L219 | L220 L221 L222 L223 | L224 L225 L226 L227 | L228 L229 L230 L231 | L232 L233 L234 L235 | L236 L237 L238 L239 | L240 L241 L242 L243 | L244 L245 L246 L247 | L248 L249 L250 L251 | L252 L253 L254 L255 | L256 L257 L258 L259 | L260 L261 L262 L263 | L264 L265 L266 L267 | L268 L269 L270 L271 | L272 L273 L274 L275 | L276 L277 L278 L279 | L280 L281 L282 L283 | L284 L285 L286 L287 | L288 L289 L290 L291 | L292 L293 L294 L295 | L296 L297 L298 L299 | L300 L301 L302 L303 | L304 L305 L306 L307 | L308 L309 L310 L311 | L312 L313 L314 L315 | L316 L317 L318 L319 | L320 L321 L322 L323 | L324 L325 L326 L327 | L328 L329 L330 L331 | L332 L333 L334 L335 | L336 L337 L338 L339 | L340 L341 L342 L343 | L344 L345 L346 L347 | L348 L349 L350 L351 | L352 L353 L354 L355 | L356 L357 L358 L359 | L360 L361 L362 L363 | L364 L365 L366 L367 | L368 L369 L370 L371 | L372 L373 L374 L375 | L376 L377 L378 L379 | L380 L381 L382 L383 | L384 L385 L386 L387 | L388 L389 L390 L391 | L392 L393 L394 L395 | L396 L397 L398 L399 | L400 L401 L402 L403 | L404 L405 L406 L407 | L408 L409 L410 L411 | L412 L413 L414 L415 | L416 L417 L418 L419 | L420 L421 L422 L423 | L424 L425 L426 L427 | L428 L429 L430 L431 | L432 L433 L434 L435 | L436 L437 L438 L439 | L440 L441 L442 L443 | L444 L445 L446 L447 | L448 L449 L450 L451 | L452 L453 L454 L455 | L456 L457 L458 L459 | L460 L461 L462 L463 | L464 L465 L466 L467 | L468 L469 L470 L471 | L472 L473 L474 L475 | L476 L477 L478 L479 | L480 L481 L482 L483 | L484 L485 L486 L487 | L488 L489 L490 L491 | L492 L493 L494 L495 | L496 L497 L498 L499 | L500 L501 L502 L503 | L504 L505 L506 L507 | L508 L509 L510 L511 | L512 L513 L514 L515 | L516 L517 L518 L519 | L520 L521 L522 L523 | L524 L525 L526 L527 | L528 L529 L530 L531 | L532 L533 L534 L535 | L536 L537 L538 L539
